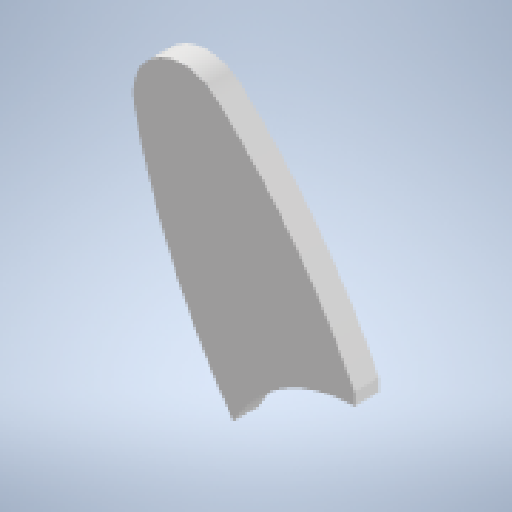
# Autodesk Inventor part: bunny ears
Saved by Autodesk Inventor 2024.2 (Build 282272000, 272)
## iProperties
Created: 2025-12-17
Part Number: bunny ears
Material: Generic
Document SubType Name: Modeling
Designer: David Toler II
Density: 1 g/cm^3
Appearance: Default
Author: David Toler II
Autodesk Inventor part; units mm, degrees
ref_plane "YZ Plane" through (0, 0, 0) normal (1, 0, 0) x (0, 1, 0)
ref_plane "XZ Plane" through (0, 0, 0) normal (0, 1, 0) x (-1, 0, 0)
ref_plane "XY Plane" through (0, 0, 0) normal (0, 0, 1) x (1, 0, 0)
sketch "Sketch1" plane through (0, 0, 0) normal (0, 0, 1) x (1, 0, 0)
  circle A0 centre (0, 0) radius 12.7
  line L0 (0, 0) -> (-43.9941, 76.2)
  line L1 (-43.9941, 76.2) -> (43.9941, 76.2)
  line L2 (43.9941, 76.2) -> (0, 0)
  line L3 (0, 0) -> (0, 76.2)
  circle A1 centre (-43.9941, 76.2) radius 12.7
  circle A2 centre (43.9941, 76.2) radius 12.7
  arc A3 (-56.3878, 73.4276) -> (-8.5978, -9.347) centre (99.6489, 108.3323) ccw
  arc A4 (12.3937, 2.7724) -> (-35.3963, 85.547) centre (-143.6429, -32.1323) ccw
  arc A5 (8.5978, -9.347) -> (56.3878, 73.4276) centre (-99.6489, 108.3323) ccw
  arc A6 (35.3963, 85.547) -> (-12.3937, 2.7724) centre (143.6429, -32.1323) ccw
  circle A7 centre (0, 0) radius 38.1
  circle A8 centre (0, 0) radius 34.925
  point P0 (-30.9793, 16.1257)
  point P1 (30.9793, 16.1257)
  point P2 (56.3878, 73.4276)
  point P3 (0, 38.0993)
  dimension "d2" = 25.4
  dimension "d3" = 25.4
  dimension "d0" = 76.2
  dimension "d1" = 60
  dimension "d4" = 25.4
  dimension "d5" = 159.893
  dimension "d6" = 76.2
  dimension "d7" = 3.175
  constraints: 9 symmetric about line, 8 end point, 8 point on circle, 7 centre point, 5 coincident, 1 horizontal, 1 midpoint, 1 perpendicular, 11 other
  measures "d0" distance from line of point (0, 0) L1
  measures "d1" angle of L2 L0
  measures "d4" diameter of A2
  measures "d5" radius of A3
  measures "d6" diameter of A7
  measures "d7" radial gap between concentric circles of A7 A8
extrude "Extrusion1" add sketch "Sketch1" along normal blind 6.35 contours A8 L2 A7 A5 | A8 A4 A7 L2 | A8 L3 A4 | A3 A7 L0 A8 | A7 L2 A2 A5 | A8 A6 L3 | A7 A6 L1 A2 L2 | A7 L0 A1 L1 A4 | A6 A8 L0 A7 | A3 A1 L0 A7 | A2 L2 L1 | A2 L1 L2 | L1 A1 A4 | A6 A2 L1 | A1 L1 L0 | A1 L0 L1
sketch "Sketch2" plane through (0, 0, 6.35) normal (0, 0, 1) x (1, 0, 0)
  arc A0 (-56.3878, 73.4276) -> (-30.9793, 16.1257) centre (99.6489, 108.3323) ccw projected
  arc A1 (30.9793, 16.1257) -> (-30.9793, 16.1257) centre (0, 0) ccw projected
  arc A2 (30.9793, 16.1257) -> (56.3878, 73.4276) centre (-99.6489, 108.3323) ccw projected
  arc A3 (56.3878, 73.4276) -> (35.3963, 85.547) centre (43.9941, 76.2) ccw projected
  arc A4 (35.3963, 85.547) -> (0, 38.0993) centre (143.6429, -32.1323) ccw projected
  arc A5 (0, 38.0993) -> (-35.3963, 85.547) centre (-143.6429, -32.1323) ccw projected
  arc A6 (-35.3963, 85.547) -> (-56.3878, 73.4276) centre (-43.9941, 76.2) ccw projected
  line L0 (0, 38.0993) -> (0, 34.925)
  constraints: 2 end point, 1 point on circle
extrude "Extrusion2" cut sketch "Sketch2" against normal through all contours L0 A4 A3 A2 A1
body "Solid1"
